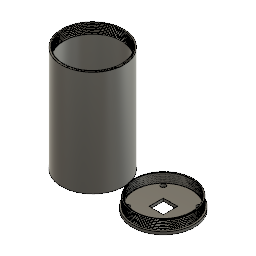
Znicz1 v4 (Autodesk Fusion 360 design; units mm, degrees)
Autodesk Fusion 360 part; units mm, degrees
sketch "Sketch1" plane through (0, 0, 0) normal (0, 1, 0) x (1, 0, 0)
  circle A0 centre (0, 0) radius 33
  dimension "d1" = 66
  measures "d1" diameter of A0
extrude "Extrude1" add sketch "Sketch1" along normal blind 112 makes body 1
sketch "Sketch2" plane through (0, 112, 0) normal (0, 1, 0) x (-1, 0, 0)
  circle A0 centre (0, 0) radius 33
  circle A1 centre (0, 0) radius 31.5
  dimension "d4" = 63
  measures "d4" diameter of A1
extrude "Extrude2" cut sketch "Sketch2" against normal blind 109 contours A1 bodies 1
thread "Thread1" "ISO Metric profile 63.0 M63x1.5 6H" major diameter 63.2143 minor diameter 61.5262 pitch 1.5 angle 60 modelled right hand crest width 0.1875 on face at (-31.4608, 39.3333, -1.5701) from (0, 112, 0) to (0, 102, 0) crest through (-30.7631, 112.8438, 0) on bodies 1
sketch "Sketch3" plane through (0, 3, 0) normal (0, 1, 0) x (-1, 0, 0)
  circle A0 centre (0, 0) radius 30.7631
  circle A1 centre (-75, 0) radius 33
  dimension "d9" = 66
  measures "d9" diameter of A1
extrude "Extrude3" add sketch "Sketch3" along normal blind 3 separate body contours A1 makes body 2
sketch "Sketch4" plane through (0, 6, 0) normal (0, 1, 0) x (-1, 0, 0)
  circle A0 centre (-75, 0) radius 33
  circle A1 centre (-75, 0) radius 31.5
  circle A2 centre (-75, 0) radius 30
  dimension "d12" = 63
  measures "d12" diameter of A1
extrude "Extrude4" add sketch "Sketch4" along normal blind 10 contours A1 bodies 2
thread "Thread2" "ISO Metric profile 63.0 M63x1.5 6g" major diameter 62.85 minor diameter 61.1269 pitch 1.5 angle 60 modelled right hand crest width 0.1875 on face at (43.5392, 12.6667, -1.5701) crest through (43.575, 5.9063, 0) on bodies 2
sketch "Sketch5" plane through (0, 3, 0) normal (0, -1, 0) x (1, 0, 0)
  circle A0 centre (75, 0) radius 33
  line L0 (94, 19) -> (56, 19)
  line L1 (56, 19) -> (56, -19)
  line L2 (56, -19) -> (94, -19)
  line L3 (94, -19) -> (94, 19)
  line L4 (94, 19) -> (56, -19) construction
  line L5 (56, 19) -> (94, -19) construction
  circle A1 centre (56, 19) radius 2.5
  circle A2 centre (94, 19) radius 2.5
  circle A3 centre (56, -19) radius 2.5
  circle A4 centre (94, -19) radius 2.5
  dimension "d15" = 5
  dimension "d16" = 5
  dimension "d17" = 5
  dimension "d18" = 5
  measures "d15" diameter of A1
  measures "d16" diameter of A2
  measures "d17" diameter of A3
  measures "d18" diameter of A4
extrude "Extrude5" cut sketch "Sketch5" against normal blind 12 contours L0 L1 A1 | L0 L1 A1 | L0 L3 A2 | L0 L3 A2 | L1 L2 A3 | L1 L2 A3 | L2 L3 A4 | L2 L3 A4 bodies 2
move_body "Move1" bodies 2 to x (1, 0, 0) y (0, 1, 0) z (0, 0, 1) at (0, -3, 0)
sketch "Sketch6" plane through (0, 3, 0) normal (0, 1, 0) x (-1, 0, 0)
  circle A0 centre (-56, 19) radius 2.5
  circle A1 centre (-94, 19) radius 2.5
  circle A2 centre (-56, -19) radius 2.5
  circle A3 centre (-94, -19) radius 2.5
  circle A4 centre (-75, 0) radius 30
  line L0 (-67.5, -7.5) -> (-82.5, -7.5)
  line L1 (-82.5, -7.5) -> (-82.5, 7.5)
  line L2 (-82.5, 7.5) -> (-67.5, 7.5)
  line L3 (-67.5, 7.5) -> (-67.5, -7.5)
  line L4 (-67.5, -7.5) -> (-82.5, 7.5) construction
  line L5 (-82.5, -7.5) -> (-67.5, 7.5) construction
  dimension "d21" = 15
  dimension "d22" = 15
extrude "Extrude6" cut sketch "Sketch6" against normal blind 3 contours L0 L1 L2 L3 bodies 2
sketch "Sketch7" plane through (0, 0, 0) normal (0, 0, 1) x (1, 0, 0)
  line L0 (-33.0685, 71.5) -> (33.0685, 71.5)
  line L1 (33.0685, 71.5) -> (33.0685, 68.5)
  line L2 (33.0685, 68.5) -> (-33.0685, 68.5)
  line L3 (-33.0685, 68.5) -> (-33.0685, 71.5)
  line L4 (-33.0685, 71.5) -> (33.0685, 68.5) construction
  line L5 (33.0685, 71.5) -> (-33.0685, 68.5) construction
  dimension "d25" = 66.1369
  dimension "d26" = 3
extrude "Extrude7" add sketch "Sketch7" along normal mid plane 66 bodies 1
delete_face "DeleteFace1" 2 faces at (-27.1049, 71.5, -25.922) (26.5395, 71.5, 26.5167) on bodies 1
sketch "Sketch8" plane through (0, 71.5, 0) normal (0, 1, 0) x (-1, 0, 0)
  circle A0 centre (0, 0) radius 30.7631
  line L0 (0, -30.7631) -> (30.7631, 0)
  line L1 (30.7631, 0) -> (0, 30.7631)
  line L2 (0, 30.7631) -> (-30.7631, 0)
  line L3 (-30.7631, 0) -> (0, -30.7631)
extrude "Extrude8" cut sketch "Sketch8" against normal blind 14 contours A0 L0 | L0 L1 L2 L3 | A0 L2 bodies 1
